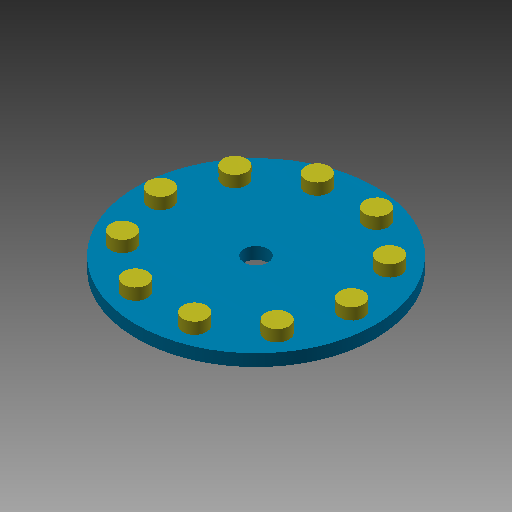
# Autodesk Inventor part: 180219-Base
Saved by Autodesk Inventor 2019 (Build 230136000, 136)
## iProperties
Created: 2018-02-21
Part Number: 180219-Base
Material: Stahl, Legierung
Document SubType Name: Modeling
Designer: Normal
Mass: 329.082 g
Surface Area: 187.716 cm^2
Volume: 42.5721 cm^3
Density: 7.73 g/cm^3
Appearance: Kanariengelb
Author: Normal
Autodesk Inventor part; units mm, degrees
ref_plane "YZ Plane" through (0, 0, 0) normal (1, 0, 0) x (0, 1, 0)
ref_plane "XZ Plane" through (0, 0, 0) normal (0, 1, 0) x (-1, 0, 0)
ref_plane "XY Plane" through (0, 0, 0) normal (0, 0, 1) x (1, 0, 0)
derived "180219-Master.ipt"
sketch "Skizze1" plane through (0, 0, 0) normal (0, 0, 1) x (1, 0, 0)
  circle A0 centre (0, 0) radius 40
  circle A1 centre (40, 0) radius 5
  line L0 (0, 0) -> (-2, 0)
  circle A2 centre (32.3607, 23.5114) radius 5
  circle A3 centre (12.3607, 38.0423) radius 5
  circle A4 centre (-12.3607, 38.0423) radius 5
  circle A5 centre (-32.3607, 23.5114) radius 5
  circle A6 centre (-40, 0) radius 5
  circle A7 centre (-32.3607, -23.5114) radius 5
  circle A8 centre (-12.3607, -38.0423) radius 5
  circle A9 centre (12.3607, -38.0423) radius 5
  circle A10 centre (32.3607, -23.5114) radius 5
  circle A11 centre (0, 0) radius 36
  circle A12 centre (40, 0) radius 4
  circle A13 centre (0, 0) radius 5
  circle A14 centre (-2, 0) radius 10
  point P0 (42, 0)
sketch "Skizze2" plane through (0, 0, 0) normal (0, 0, 1) x (1, 0, 0)
  line L0 (0, 0) -> (9.3969, 3.4202) construction
  line L1 (0, 0) -> (9.3969, -3.4202) construction
  line L2 (0, 0) -> (42, 0) construction
  arc A0 (9.3969, -3.4202) -> (9.3969, 3.4202) centre (0, 0) ccw
  line L3 (9.3969, -3.4202) -> (31.0099, -11.2867)
  line L4 (9.3969, 3.4202) -> (31.0099, 11.2867)
  arc A1 (9.3969, 3.4202) -> (9.3969, -3.4202) centre (0, 0) ccw
  spline S0 degree 3 poles (31.0099, -11.2867) (31.0596, -11.15) (31.1671, -10.8796) (31.3182, -10.5552) (31.4787, -10.2448) (31.613, -10.0088) (31.785, -9.7307) (31.9245, -9.522) (32.1331, -9.2293) (32.3392, -8.963) (32.6366, -8.6062) (32.8861, -8.328) (33.1792, -8.0137) (33.4001, -7.7834) (33.6628, -7.5104) (33.8642, -7.3001) (34.1081, -7.0396) (34.2982, -6.8306) (34.5315, -6.5635) (34.7149, -6.3435) (34.9406, -6.0573) (35.1182, -5.8183) (35.3356, -5.505) (35.5054, -5.2423) (35.752, -4.8288) (35.9864, -4.3891) (36.3063, -3.681) (36.55, -3.0022) (36.7886, -2.1037) (36.9214, -1.3516) (37.0056, -0.3893) (37.0056, 0.3893) (36.9214, 1.3516) (36.7886, 2.1037) (36.55, 3.0022) (36.3063, 3.681) (35.9864, 4.3891) (35.752, 4.8288) (35.5054, 5.2423) (35.3356, 5.505) (35.1182, 5.8183) (34.9406, 6.0573) (34.7149, 6.3435) (34.5315, 6.5635) (34.2982, 6.8306) (34.1081, 7.0396) (33.8642, 7.3001) (33.6628, 7.5104) (33.4001, 7.7834) (33.1792, 8.0137) (32.8861, 8.328) (32.6366, 8.6062) (32.3392, 8.963) (32.1331, 9.2293) (31.9245, 9.522) (31.785, 9.7307) (31.613, 10.0088) (31.4787, 10.2448) (31.3182, 10.5552) (31.1671, 10.8796) (31.0596, 11.15) (31.0099, 11.2867) knots -0.349066 -0.349066 -0.349066 -0.349066 -0.341794 -0.334521 -0.330885 -0.323613 -0.319977 -0.312705 -0.309069 -0.29816 -0.290888 -0.276344 -0.269072 -0.254527 -0.247255 -0.232711 -0.225438 -0.210894 -0.203622 -0.189077 -0.181805 -0.167261 -0.159989 -0.145444 -0.138172 -0.116355 -0.101811 -0.072722 -0.058178 -0.029089 -0.014544 0.014544 0.029089 0.058178 0.072722 0.101811 0.116355 0.138172 0.145444 0.159989 0.167261 0.181805 0.189077 0.203622 0.210894 0.225438 0.232711 0.247255 0.254527 0.269072 0.276344 0.290888 0.29816 0.309069 0.312705 0.319977 0.323613 0.330885 0.334521 0.341794 0.349066 0.349066 0.349066 0.349066
  spline S1 degree 3 poles (35.7083, -12.9968) (35.9684, -12.2823) (36.5997, -11.6816) (37.4946, -10.7372) (38.384, -9.7987) (39.5052, -8.4934) (40.3973, -6.7316) (41.3238, -4.9021) (41.9604, -2.5931) (41.9981, -0.24) (42.0346, 2.0396) (41.5095, 4.3183) (40.6653, 6.1739) (39.8297, 8.0104) (38.7163, 9.4155) (37.7885, 10.423) (36.8593, 11.4319) (36.1466, 12.0655) (35.8121, 12.7523) (35.773, 12.8327) (35.7385, 12.9139) (35.7083, 12.9968) knots -0.349066 -0.349066 -0.349066 -0.349066 -0.235021 -0.235021 -0.235021 -0.121688 -0.121688 -0.121688 -0.004 -0.004 -0.004 0.110008 0.110008 0.110008 0.222841 0.222841 0.222841 0.335844 0.335844 0.335844 0.349066 0.349066 0.349066 0.349066
  circle A2 centre (22.5, 0) radius 4
  circle A3 centre (22.5, 0) radius 6
sketch "Skizze4" plane through (0, 0, 0) normal (0, 0, 1) x (1, 0, 0)
  circle A0 centre (0, 0) radius 50
  circle A1 centre (40, 0) radius 5 projected
  dimension "d1" = 5
  constraints: 1 centre point, 1 coincident
extrude "Extrusion1" add sketch "Skizze4" along normal blind 5 contours A0 | A1
extrude "Extrusion2" cut sketch "Skizze1" along normal through all contours A13
extrude "Extrusion3" add sketch "Skizze1" along normal blind 9.8 contours A0 A12 | A0 A12 | A12 A11 A1 A0 | A0 A1 A12 | A0 A1 A11 A12 | A11 A1
thicken "Verdickung1" operation cut thickness 0.05 both sides no extend neighbours no toward (-0.9870503, -0.1604113, 0) faces at (44.9353, 0.8021, 6.6)
pattern_circular "Runde Anordnung1" count 10 over 360 about axis through (0, 0, 0) along (0, 0, 1) of "Extrusion3", "Verdickung1"
